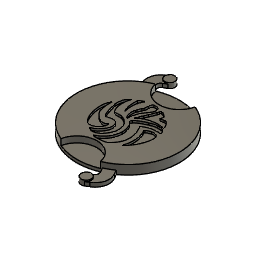
Deckbox - Key - Bant (Autodesk Fusion 360 design; units mm, degrees)
Autodesk Fusion 360 part; units mm, degrees
sketch "Sketch1" plane through (0, 0, 0) normal (0, 1, 0) x (1, 0, 0)
  circle A0 centre (0, 0) radius 25.4
  line L0 (19.5918, -28.934) -> (-15.2617, 31.434)
  line L1 (-19.5918, 28.934) -> (15.2617, -31.434)
  line L2 (0, -25.4) -> (0, 25.4) construction
  line L3 (0, 0) -> (25.4, 0) construction
  line L4 (-19.5918, 28.934) -> (-15.2617, 31.434)
  line L5 (15.2617, -31.434) -> (19.5918, -28.934)
  line L6 (17.4268, -30.184) -> (-17.4268, 30.184) construction
  line L7 (-2.1651, -1.25) -> (2.1651, 1.25) construction
  line L8 (19.5918, -28.934) -> (11.7976, -33.434)
  line L9 (11.7976, -33.434) -> (9.2976, -29.1039)
  line L10 (9.2976, -29.1039) -> (17.0918, -24.6039)
  line L11 (17.0918, -24.6039) -> (19.5918, -28.934)
  circle A1 centre (10.5476, -31.269) radius 2.5
  circle A2 centre (0, 0) radius 35.5
  line L12 (-19.5918, 28.934) -> (-17.0918, 24.6039)
  line L13 (-17.0918, 24.6039) -> (-9.2976, 29.1039)
  line L14 (-9.2976, 29.1039) -> (-11.7976, 33.434)
  line L15 (-11.7976, 33.434) -> (-19.5918, 28.934)
  circle A3 centre (-10.5476, 31.269) radius 2.5
  point P0 (-12.5, 21.6506)
  point P1 (12.5, -21.6506)
  dimension "d1" = 50.8
  dimension "d42" = 5
  dimension "d45" = 5
  dimension "d46" = 71
  dimension "d47" = 60
  dimension "d48" = 4
  dimension "d51" = 5
  constraint coincident A0.centre L3.start
  constraint coincident A0 L2.start
  constraint coincident A0 L2.end
  constraint coincident A0.centre L2
  constraint coincident A0 L3.end
  constraint horizontal L3
  constraint perpendicular L0 L4
  constraint perpendicular L0 L5
  constraint perpendicular L1 L4
  constraint midpoint L5 L6.start
  constraint midpoint L4 L6.end
  constraint perpendicular L4 L6
  constraint midpoint L1 L7.start
  constraint midpoint L0 L7.end
  constraint midpoint L6 A0.centre
  constraint perpendicular L8 L9
  constraint parallel L8 L10
  constraint parallel L9 L11
  constraint perpendicular L0 L8
  constraint midpoint L9 A1.centre
  constraint tangent L10 A1
  constraint concentric A0 A2
  constraint tangent A1 A2
  constraint perpendicular L12 L13
  constraint parallel L12 L14
  constraint parallel L13 L15
  constraint coincident L1 L12.end
  constraint midpoint L14 A3.centre
  constraint tangent L13 A3
  constraint tangent A2 A3
  measures "d1" diameter of A0
  measures "d42" distance of L0 L1
  measures "d45" diameter of A1
  measures "d46" diameter of A2 A0.centre
  measures "d47" angle of L3 L6
  measures "d48" distance of L1 A1.centre
  measures "d51" diameter of A3
extrude "Extrude1" add sketch "Sketch1" along normal blind 4.5 contours A0 L0 | A0 L0 L1 | A0 L1
extrude "Extrude2" add sketch "Sketch1" along normal blind 1.9 contours A0 L0 | A0 L0 L1 | A0 L0 L1 L13 | A0 L0 L1 L10 | A0 L1 | L0 L1 L4 L12 L13 L15 | L0 L13 L15 A3 | L0 L1 L5 L8 L10 L11 | L14 A3 | L14 A3 | L1 L8 L10 A1 | L9 A1 | L9 A1
extrude "Extrude3" add sketch "Sketch1" along normal blind 2.5 contours L14 A3 | L14 A3 | L9 A1 | L9 A1
sketch "Sketch2" plane through (0, 4.5, 0) normal (0, 1, 0) x (-1, 0, 0)
  circle A0 centre (0, 0) radius 25.4
  circle A1 centre (0, -25.4) radius 10
  circle A2 centre (0, 25.4) radius 10
  line L0 (0, -25.4) -> (0, 25.4) construction
  dimension "d18" = 20
  dimension "d19" = 20
  constraint coincident A0 A1.centre
  constraint coincident A0 A2.centre
  constraint coincident A1.centre L0.start
  constraint coincident A2.centre L0.end
  constraint coincident A0.centre L0
  constraint vertical L0
  measures "d18" diameter of A1
  measures "d19" diameter of A2
extrude "Extrude4" cut sketch "Sketch2" against normal blind 3 contours A0 A2 | A0 A1 picked at (-1.832, 22.0709) picked at (1.832, -22.0709)
fillet "Fillet6" radius 2 2 edges at (12.7617, 0.95, 27.1039) (-12.7617, 0.95, -27.1039)
fillet "Fillet7" radius 7 2 edges at (19.5918, 0.95, 28.934) (-19.5918, 0.95, -28.934)
sketch "Sketch4" plane through (0, 4.5, 0) normal (0, 1, 0) x (-1, 0, 0)
  arc A0 (-9.8043, 23.4315) -> (-9.8043, -23.4315) centre (0, 0) ccw
  arc A1 (9.8043, -23.4315) -> (-9.8043, -23.4315) centre (0, -25.4) ccw
  arc A2 (9.8043, -23.4315) -> (9.8043, 23.4315) centre (0, 0) ccw
  spline S0 degree 3 poles (1.1102, -13.9365) (1.7648, -13.8115) (1.9245, -13.4736) (2.0071, -12.0381) knots 0 0 0 0 1 1 1 1
  spline S1 degree 3 poles (2.0071, -12.0381) (2.0518, -11.2614) (2.1651, -10.4715) (2.2652, -10.2392) knots 0 0 0 0 1 1 1 1
  spline S2 degree 3 poles (2.2652, -10.2392) (2.2894, -10.183) (2.4399, -9.8609) (2.5996, -9.5236) knots 0 0 0 0 1 1 1 1
  spline S3 degree 3 poles (2.5996, -9.5236) (3.0226, -8.6301) (3.2054, -8.1919) (3.3353, -7.7602) knots 0 0 0 0 1 1 1 1
  spline S4 degree 3 poles (3.3353, -7.7602) (3.3988, -7.5493) (3.4831, -7.2773) (3.5228, -7.1556) knots 0 0 0 0 1 1 1 1
  spline S5 degree 3 poles (3.5228, -7.1556) (4.0509, -5.5359) (3.662, -3.3705) (2.6052, -2.0463) knots 0 0 0 0 1 1 1 1
  spline S6 degree 3 poles (2.6052, -2.0463) (2.1621, -1.4911) (2.1825, -1.4853) (2.1423, -2.176) knots 0 0 0 0 1 1 1 1
  spline S7 degree 3 poles (2.1423, -2.176) (1.9767, -5.0213) (1.385, -6.5935) (-0.4784, -9.1402) knots 0 0 0 0 1 1 1 1
  spline S8 degree 3 poles (-0.4784, -9.1402) (-1.5227, -10.5675) (-1.7724, -11.12) (-1.7721, -12.0025) knots 0 0 0 0 1 1 1 1
  spline S9 degree 3 poles (-1.7721, -12.0025) (-1.7718, -12.99) (-1.4169, -13.8064) (-0.9301, -13.9395) knots 0 0 0 0 1 1 1 1
  spline S10 degree 3 poles (-0.9301, -13.9395) (-0.6853, -14.0064) (0.7552, -14.0043) (1.1102, -13.9365) knots 0 0 0 0 1 1 1 1
  spline S11 degree 3 poles (5.0501, -13.2068) (5.7804, -12.9161) (6.7744, -12.4301) (7.0495, -11.7289) knots 0 0 0 0 1 1 1 1
  spline S12 degree 3 poles (7.0495, -11.7289) (7.3052, -9.4302) (7.0314, -6.2402) (5.877, -4.4378) knots 0 0 0 0 1 1 1 1
  line L0 (5.877, -4.4378) -> (5.777, -4.31)
  line L1 (5.777, -4.31) -> (5.8085, -4.4418)
  spline S13 degree 3 poles (5.8085, -4.4418) (6.1088, -5.7005) (6.1977, -6.5848) (6.201, -8.348) knots 0 0 0 0 1 1 1 1
  spline S14 degree 3 poles (6.201, -8.348) (6.1393, -9.6884) (5.6874, -12.1521) (4.8697, -12.9183) knots 0 0 0 0 1 1 1 1
  spline S15 degree 3 poles (4.8697, -12.9183) (4.555, -13.2117) (4.6364, -13.3419) (5.0501, -13.2068) knots 0 0 0 0 1 1 1 1
  spline S16 degree 3 poles (-3.1327, -12.5031) (-3.0228, -12.1575) (-2.8811, -11.7368) (-2.8177, -11.5681) knots 0 0 0 0 1 1 1 1
  spline S17 degree 3 poles (-2.8177, -11.5681) (-2.5635, -10.8916) (-1.9602, -9.3702) (-1.6016, -8.5013) knots 0 0 0 0 1 1 1 1
  spline S18 degree 3 poles (-1.6016, -8.5013) (-1.2566, -7.6652) (-1.1331, -7.3737) (-0.9304, -6.9168) knots 0 0 0 0 1 1 1 1
  spline S19 degree 3 poles (-0.9304, -6.9168) (-0.7005, -6.3988) (-0.2401, -5.2994) (-0.2401, -5.2685) knots 0 0 0 0 1 1 1 1
  spline S20 degree 3 poles (-0.2401, -5.2685) (-0.2401, -5.2094) (0.221, -4.1872) (0.4075, -3.8328) knots 0 0 0 0 1 1 1 1
  spline S21 degree 3 poles (0.4075, -3.8328) (0.6691, -3.3356) (0.5757, -3.2556) (0.1869, -3.644) knots 0 0 0 0 1 1 1 1
  spline S22 degree 3 poles (0.1869, -3.644) (0.0223, -3.8084) (-0.3423, -4.125) (-0.6235, -4.3475) knots 0 0 0 0 1 1 1 1
  spline S23 degree 3 poles (-0.6235, -4.3475) (-2.6101, -6.3099) (-6.619, -6.8669) (-8.7795, -6.789) knots 0 0 0 0 1 1 1 1
  spline S24 degree 3 poles (-8.7795, -6.789) (-9.5938, -6.7597) (-10.2837, -6.5999) (-11.043, -6.4537) knots 0 0 0 0 1 1 1 1
  spline S25 degree 3 poles (-11.043, -6.4537) (-11.5172, -6.2807) (-10.9522, -7.73) (-10.1756, -8.6785) knots 0 0 0 0 1 1 1 1
  spline S26 degree 3 poles (-10.1756, -8.6785) (-9.1154, -9.9735) (-8.6274, -10.252) (-7.8752, -9.9917) knots 0 0 0 0 1 1 1 1
  spline S27 degree 3 poles (-7.8752, -9.9917) (-7.5974, -9.8956) (-6.2437, -9.6826) (-6.1469, -9.7197) knots 0 0 0 0 1 1 1 1
  spline S28 degree 3 poles (-6.1469, -9.7197) (-6.0453, -9.7587) (-6.0444, -9.877) (-6.1449, -9.9776) knots 0 0 0 0 1 1 1 1
  spline S29 degree 3 poles (-6.1449, -9.9776) (-6.4809, -10.3135) (-6.6449, -11.1443) (-6.4236, -11.3892) knots 0 0 0 0 1 1 1 1
  spline S30 degree 3 poles (-6.4236, -11.3892) (-6.3347, -11.4876) (-6.2353, -11.6038) (-6.2028, -11.6474) knots 0 0 0 0 1 1 1 1
  spline S31 degree 3 poles (-6.2028, -11.6474) (-5.4064, -12.2123) (-4.561, -12.9579) (-3.588, -13.0981) knots 0 0 0 0 1 1 1 1
  spline S32 degree 3 poles (-3.588, -13.0981) (-3.1989, -13.212) (-3.2315, -12.8138) (-3.1327, -12.5031) knots 0 0 0 0 1 1 1 1
  spline S33 degree 3 poles (9.3795, -10.7032) (9.4554, -10.6636) (9.5689, -10.5833) (9.6319, -10.5246) knots 0 0 0 0 1 1 1 1
  spline S34 degree 3 poles (9.6319, -10.5246) (11.1499, -9.104) (11.4969, -6.9146) (11.3032, -4.8467) knots 0 0 0 0 1 1 1 1
  spline S35 degree 3 poles (11.3032, -4.8467) (11.1185, -3.8508) (9.3842, 3.0434) (8.2486, 2.8012) knots 0 0 0 0 1 1 1 1
  spline S36 degree 3 poles (8.2486, 2.8012) (6.9143, 2.3557) (4.6647, 1.8116) (3.6151, 2.622) knots 0 0 0 0 1 1 1 1
  spline S37 degree 3 poles (3.6151, 2.622) (0.3464, 5.146) (4.2821, 10.8513) (7.1841, 11.3279) knots 0 0 0 0 1 1 1 1
  spline S38 degree 3 poles (7.1841, 11.3279) (7.2614, 11.3336) (7.3682, 11.3423) (7.4214, 11.3472) knots 0 0 0 0 1 1 1 1
  spline S39 degree 3 poles (7.4214, 11.3472) (7.6985, 11.3728) (7.5397, 11.6472) (7.0571, 11.9766) knots 0 0 0 0 1 1 1 1
  spline S40 degree 3 poles (7.0571, 11.9766) (5.1961, 13.247) (2.6176, 12.2916) (0.83, 9.6694) knots 0 0 0 0 1 1 1 1
  spline S41 degree 3 poles (0.83, 9.6694) (-1.0694, 6.883) (-1.1125, 3.7051) (0.7151, 1.1846) knots 0 0 0 0 1 1 1 1
  spline S42 degree 3 poles (0.7151, 1.1846) (1.6946, -0.0491) (2.889, -0.7336) (4.2068, -1.1853) knots 0 0 0 0 1 1 1 1
  spline S43 degree 3 poles (4.2068, -1.1853) (5.7092, -1.7361) (7.5723, -0.7103) (8.299, -1.7076) knots 0 0 0 0 1 1 1 1
  spline S44 degree 3 poles (8.299, -1.7076) (9.639, -3.4317) (9.9297, -6.2219) (9.724, -8.0397) knots 0 0 0 0 1 1 1 1
  spline S45 degree 3 poles (9.724, -8.0397) (9.6966, -8.2374) (9.6645, -8.4681) (9.6527, -8.5524) knots 0 0 0 0 1 1 1 1
  spline S46 degree 3 poles (9.6527, -8.5524) (9.6114, -8.8474) (9.5283, -9.2208) (9.3964, -9.7025) knots 0 0 0 0 1 1 1 1
  spline S47 degree 3 poles (9.3964, -9.7025) (9.3234, -9.9695) (9.2419, -10.2685) (9.2154, -10.3669) knots 0 0 0 0 1 1 1 1
  spline S48 degree 3 poles (9.2154, -10.3669) (9.1113, -10.7532) (9.1462, -10.8249) (9.3795, -10.7032) knots 0 0 0 0 1 1 1 1
  spline S49 degree 3 poles (-11.0331, -5.8442) (-10.9773, -5.8371) (-9.3356, -6.0248) (-8.4772, -5.9978) knots 0 0 0 0 1 1 1 1
  spline S50 degree 3 poles (-8.4772, -5.9978) (-7.3091, -6.0092) (-6.1289, -5.5058) (-5.2116, -5.1254) knots 0 0 0 0 1 1 1 1
  spline S51 degree 3 poles (-5.2116, -5.1254) (-3.3661, -4.3569) (-1.1291, -3.2046) (-0.2049, -1.9794) knots 0 0 0 0 1 1 1 1
  spline S52 degree 3 poles (-0.2049, -1.9794) (0.3045, -1.3042) (0.3196, -1.1165) (0.1093, -0.9281) knots 0 0 0 0 1 1 1 1
  spline S53 degree 3 poles (0.1093, -0.9281) (0.0204, -0.8484) (-0.1777, -0.6682) (-0.331, -0.5277) knots 0 0 0 0 1 1 1 1
  spline S54 degree 3 poles (-0.331, -0.5277) (-1.6356, 0.6689) (-2.562, 3.2359) (-2.4707, 5.4014) knots 0 0 0 0 1 1 1 1
  spline S55 degree 3 poles (-2.4707, 5.4014) (-2.1561, 9.2614) (-0.3167, 12.0514) (3.1462, 13.7893) knots 0 0 0 0 1 1 1 1
  spline S56 degree 3 poles (3.1462, 13.7893) (3.6495, 14.0355) (3.5573, 14.0767) (2.2389, 14.1936) knots 0 0 0 0 1 1 1 1
  spline S57 degree 3 poles (2.2389, 14.1936) (0.4794, 14.3498) (-1.0006, 14.2388) (-2.5658, 13.8336) knots 0 0 0 0 1 1 1 1
  spline S58 degree 3 poles (-2.5658, 13.8336) (-3.9258, 13.4815) (-5.7033, 11.4179) (-6.4926, 9.2744) knots 0 0 0 0 1 1 1 1
  spline S59 degree 3 poles (-6.4926, 9.2744) (-7.4096, 6.7845) (-7.1301, 3.8102) (-5.7054, 0.8976) knots 0 0 0 0 1 1 1 1
  spline S60 degree 3 poles (-5.7054, 0.8976) (-5.4584, 0.3154) (-5.1311, -0.2738) (-4.8403, -0.7832) knots 0 0 0 0 1 1 1 1
  spline S61 degree 3 poles (-4.8403, -0.7832) (-4.7456, -0.9519) (-4.6436, -1.1079) (-4.6136, -1.1299) knots 0 0 0 0 1 1 1 1
  spline S62 degree 3 poles (-4.6136, -1.1299) (-4.4652, -1.2387) (-5.6792, -2.1741) (-6.4503, -2.5451) knots 0 0 0 0 1 1 1 1
  spline S63 degree 3 poles (-6.4503, -2.5451) (-7.9562, -3.2695) (-10.3768, -3.6175) (-12.1994, -3.3716) knots 0 0 0 0 1 1 1 1
  spline S64 degree 3 poles (-12.1994, -3.3716) (-12.6623, -3.3091) (-12.7117, -3.3383) (-12.7117, -3.6749) knots 0 0 0 0 1 1 1 1
  spline S65 degree 3 poles (-12.7117, -3.6749) (-12.7268, -4.4443) (-12.071, -5.1416) (-11.485, -5.6478) knots 0 0 0 0 1 1 1 1
  spline S66 degree 3 poles (-11.485, -5.6478) (-11.3607, -5.7551) (-11.0894, -5.819) (-11.0331, -5.8442) knots 0 0 0 0 1 1 1 1
  spline S67 degree 3 poles (13.0494, -4.9824) (15.2998, -0.7388) (13.5971, 6.0633) (10.9026, 9.2615) knots 0 0 0 0 1 1 1 1
  spline S68 degree 3 poles (10.9026, 9.2615) (10.1069, 10.0726) (9.8454, 10.1904) (8.8415, 10.189) knots 0 0 0 0 1 1 1 1
  spline S69 degree 3 poles (8.8415, 10.189) (6.617, 10.1862) (4.8938, 8.908) (4.3579, 6.8633) knots 0 0 0 0 1 1 1 1
  spline S70 degree 3 poles (4.3579, 6.8633) (4.1055, 5.9003) (4.1212, 4.8605) (4.3825, 5.2335) knots 0 0 0 0 1 1 1 1
  spline S71 degree 3 poles (4.3825, 5.2335) (6.9277, 8.15) (11.4873, 3.2757) (12.0457, 1.8235) knots 0 0 0 0 1 1 1 1
  spline S72 degree 3 poles (12.0457, 1.8235) (12.6414, 0.1193) (12.8778, -1.3515) (12.9308, -3.6839) knots 0 0 0 0 1 1 1 1
  spline S73 degree 3 poles (12.9308, -3.6839) (12.948, -4.4359) (12.9816, -5.0512) (13.0056, -5.0512) knots 0 0 0 0 1 1 1 1
  spline S74 degree 3 poles (13.0056, -5.0512) (13.0296, -5.0512) (13.0494, -5.0202) (13.0494, -4.9824) knots 0 0 0 0 1 1 1 1
  spline S75 degree 3 poles (-9.7036, -1.9821) (-8.8584, -1.7219) (-8.1199, -1.3816) (-7.5365, -0.8412) knots 0 0 0 0 1 1 1 1
  spline S76 degree 3 poles (-7.5365, -0.8412) (-7.2519, -0.5768) (-7.242, -0.5196) (-7.447, -0.3232) knots 0 0 0 0 1 1 1 1
  spline S77 degree 3 poles (-7.447, -0.3232) (-9.1564, 2.5892) (-9.655, 8.0382) (-8.2883, 10.5221) knots 0 0 0 0 1 1 1 1
  spline S78 degree 3 poles (-8.2883, 10.5221) (-8.1686, 10.6419) (-8.1892, 10.9983) (-8.3159, 10.9983) knots 0 0 0 0 1 1 1 1
  spline S79 degree 3 poles (-8.3159, 10.9983) (-8.5356, 10.9076) (-8.7081, 10.6495) (-8.8584, 10.515) knots 0 0 0 0 1 1 1 1
  spline S80 degree 3 poles (-8.8584, 10.515) (-11.3564, 8.2865) (-13.5289, 3.0985) (-13.252, 0.0233) knots 0 0 0 0 1 1 1 1
  spline S81 degree 3 poles (-13.252, 0.0233) (-13.1108, -1.5447) (-11.5334, -2.4362) (-9.7036, -1.9821) knots 0 0 0 0 1 1 1 1
extrude "Extrude6" cut sketch "Sketch4" against normal blind 1
named bodies: "Deckbox - Key - Bant"
